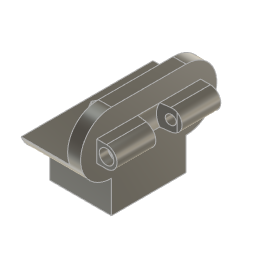
1-4-20mount (Autodesk Fusion 360 design; units mm, degrees)
Autodesk Fusion 360 part; units mm, degrees
note: some values were not read from the file. Set by a fixed rule: which sketch regions a step uses.
sketch "Sketch1" plane through (0, 0, 0) normal (1, 0, 0) x (0, 1, 0)
  line L0 (9.5, -9.5) -> (32.5, -9.5)
  arc A0 (32.5, -9.5) -> (32.5, 9.5) centre (32.5, 0) ccw
  line L1 (32.5, 9.5) -> (9.5, 9.5)
  arc A1 (9.5, 9.5) -> (9.5, -9.5) centre (9.5, 0) ccw
  line L2 (0, 0) -> (42, 0) construction
  dimension "d1" = 42
  dimension "d2" = 19
  constraint tangent L0 A0
  constraint tangent A0 L1
  constraint parallel L0 L1
  constraint tangent L1 A1
  constraint tangent L0 A1
  constraint midpoint A1 L2.start
  constraint midpoint A0 L2.end
  constraint horizontal L2
  constraint coincident L2.start origin
  measures "d1" distance of L2.start L2.end
  measures "d2" distance of L0 L1
extrude "Extrude1" add sketch "Sketch1" along normal blind 4
ref_plane "WorkPlane1" through (0, 5, 0) normal (0, 1, 0) x (0, 0, 1)
sketch "Sketch3" plane through (0, 5, 0) normal (0, 1, 0) x (1, 0, 0)
  line L0 (4, -9.5) -> (4, 9.5)
  line L1 (4, 0) -> (12.5887, 0) construction
  circle A0 centre (7, 0) radius 3.25
  circle A1 centre (7, 0) radius 2.25
  line L2 (7, -3.25) -> (4, -3.25)
  line L3 (7, 3.25) -> (4, 3.25)
  circle A2 centre (7, 0) radius 2
  line L4 (5.7674, -1.575) -> (8.2326, -1.575)
  line L5 (8.2326, 1.575) -> (5.7674, 1.575)
  dimension "d6" = 6.5
  dimension "d7" = 3
  dimension "d8" = 4.5
  dimension "d24" = 4
  dimension "d25" = 3.15
  constraint midpoint L0 L1.start
  constraint perpendicular L0 L1
  constraint coincident L1 A0.centre
  constraint concentric A0 A1
  constraint coincident A0 L2.start
  constraint coincident L0 L2.end
  constraint tangent A0 L2
  constraint coincident A0 L3.start
  constraint coincident L0 L3.end
  constraint tangent A0 L3
  constraint horizontal L2
  constraint horizontal L3
  constraint concentric A1 A2
  constraint coincident A2 L4.start
  constraint coincident A2 L4.end
  constraint horizontal L4
  constraint coincident A2 L5.start
  constraint coincident A2 L5.end
  constraint parallel L4 L5
  constraint equal L4 L5
  measures "d6" diameter of A0
  measures "d7" distance of L1.start A0.centre
  measures "d8" diameter of A1
  measures "d24" diameter of A2
  measures "d25" distance of L4 L5
extrude "Extrude2" add sketch "Sketch3" along normal blind 32 contours L0 A0 L2 | L0 A0 | L0 A0 L3 | A1 | A2 L4 L5 | A2 L5 | A2 L4 picked at (4.25, 0)
sketch "Sketch7" plane through (0, 0, 3.25) normal (0, 0, 1) x (-1, 0, 0)
  line L0 (-4, -5) -> (-7, -5)
  line L1 (-7, -5) -> (-7, -37)
  line L2 (-7, -37) -> (-4, -37)
  line L3 (-4, -37) -> (-4, -5)
  line L4 (-10.25, -5) -> (-7, -5)
  line L5 (-7, -5) -> (-7, -37)
  line L6 (-10.25, -37) -> (-7, -37)
  line L7 (-7, -37) -> (-7, -5)
  line L8 (-10.25, -37) -> (-10.25, -5) construction
  line L9 (-10.25, -25.04) -> (-10.25, -16.96)
  line L10 (-4, -24.39) -> (-4, -17.61)
  line L11 (-4, -17.61) -> (-4, -5) construction
  line L12 (-4, -24.39) -> (-4, -37) construction
  line L13 (-10.25, -25.04) -> (-8.75, -25.04)
  line L14 (-10.25, -16.96) -> (-8.75, -16.96)
  line L15 (-8.75, -16.96) -> (-4, -17.61)
  line L16 (-8.75, -25.04) -> (-4, -24.39)
  dimension "d15" = 8.08
  dimension "d16" = 6.78
  dimension "d44" = 1.5
  constraint coincident L6.start L8.start
  constraint coincident L4.start L8.end
  constraint coincident L3 L10.start
  constraint coincident L3 L10.end
  constraint coincident L8 L9.end
  constraint coincident L0.start L3.end
  constraint coincident L2.end L3.start
  constraint equal L11 L12
  constraint perpendicular L8 L13
  constraint perpendicular L8 L14
  constraint equal L13 L14
  constraint equal L15 L16
  measures "d15" distance of L9.start L9.end
  measures "d16" distance of L10.start L10.end
  measures "d44" distance of L9.start L13.end
extrude "Extrude3" cut sketch "Sketch7" against normal up to surface (6.5 mm away) contours L1 L3 L5 L7 L10 L15 L16 | L1 L5 L7 L9 L13 L14 L15 L16
sketch "Sketch9" plane through (0, 37, 0) normal (0, 1, 0) x (-1, 0, 0)
  arc A0 (-7, 3.25) -> (-7, -3.25) centre (-7, 0) ccw
  line L0 (-7, -3.25) -> (-4, -3.25)
  line L1 (-4, -3.25) -> (-4, 3.25)
  line L2 (-4, 3.25) -> (-7, 3.25)
  circle A1 centre (-7, 0) radius 3.25
  circle A2 centre (-7, 0) radius 2.25
hole "Hole1" at (7, 37, 0) direction (0, -1, 0) diameter 3 depth 14 tip angle 118 counterbore diameter 4.55 counterbore depth 1.5
extrude "Extrude4" cut sketch "Sketch3" along normal blind 15 contours A2 L4 L5
extrude "Extrude5" cut sketch "Sketch3" along normal blind 2.65 contours A1 | A2 L5 | A2 L4
ref_plane "WorkPlane2" through (7.125, 17.61, 0) normal (0, -1, 0) x (-1, 0, 0)
sketch "Sketch11" plane through (7.125, 17.61, 0) normal (0, -1, 0) x (1, 0, 0)
  line L0 (-0.125, 3.25) -> (-3.125, 3.25)
  line L1 (-3.125, -9.5) -> (-3.125, 9.5)
  line L2 (-0.125, -3.25) -> (-3.125, -3.25)
  line L3 (-0.125, 0) -> (-7, 0) construction
  line L4 (-3.125, 0) -> (-4, 0)
  arc A0 (-3.125, 3.25) -> (-3.125, -3.25) centre (2.4732, 0) ccw
  constraint perpendicular L1 L3
  constraint midpoint L1 L4.start
  constraint coincident L3 L4.end
  constraint perpendicular L1 L4
  constraint coincident L4.end A0
  constraint coincident L2.end A0.end
  constraint coincident L0.end A0.start
extrude "Extrude6" cut sketch "Sketch11" along normal up to surface end surface through (7, 24.8005, 3.25) normal (0.135579, -0.990767, 0) offset 0
sketch "Sketch12" plane through (0, 21, 0) normal (1, 0, 0) x (0, 1, 0)
  arc A0 (-11.5, 9.5) -> (-11.5, -9.5) centre (-11.5, 0) ccw
  line L0 (-11.5, 9.5) -> (11.5, 9.5)
  arc A1 (11.5, -9.5) -> (11.5, 9.5) centre (11.5, 0) ccw
  line L1 (11.5, -9.5) -> (-11.5, -9.5)
  line L2 (20.3318, -3.5) -> (-20.3318, -3.5)
  line L3 (-11.5, -9.5) -> (11.5, -9.5)
  dimension "d33" = 6
  constraint coincident A1 L2.start
  constraint coincident A0 L2.end
  constraint horizontal L2
  measures "d33" distance of L2 L3
extrude "Extrude7" add sketch "Sketch12" against normal blind 15 contours A0 A1 L1 L2 L3
sketch "Sketch13" plane through (0, 0, -3.5) normal (0, 0, 1) x (-1, 0, 0)
  line L0 (0, -0.6682) -> (0, -41.3318)
  line L1 (0, -41.3318) -> (15, -41.3318)
  line L2 (15, -41.3318) -> (15, -0.6682)
  line L3 (15, -0.6682) -> (0, -0.6682)
  line L4 (15, -41.3318) -> (0, -0.6682) construction
  line L5 (0, -41.3318) -> (15, -0.6682) construction
  line L6 (4.4112, -15.65) -> (1.3224, -21)
  line L7 (1.3224, -21) -> (4.4112, -26.35)
  line L8 (4.4112, -26.35) -> (10.5888, -26.35)
  line L9 (10.5888, -26.35) -> (13.6776, -21)
  line L10 (13.6776, -21) -> (10.5888, -15.65)
  line L11 (10.5888, -15.65) -> (4.4112, -15.65)
  point P0 (7.5, -21)
  dimension "d36" = 5.35
  constraint coincident L1.end L2.start
  constraint coincident L0.start L3.end
  constraint coincident L0.end L1.start
  constraint coincident L2.end L3.start
  constraint midpoint L4 P0
  constraint horizontal L11
  measures "d36" distance of P0 L11
extrude "Extrude8" cut sketch "Sketch13" against normal blind 4 contours L6 L7 L8 L9 L10 L11
hole "Hole2" at (-7.5, 21, -3.5) direction (0, 0, -1) diameter 6.756 depth 6 tip angle 118
extrude "Extrude9" add 1 faces at (1.2895, 21.0841, -9.5) along direction (0, 0, -1) blind 10
equation "d36 = ( 10.7 / 2 ) * 1 mm"
